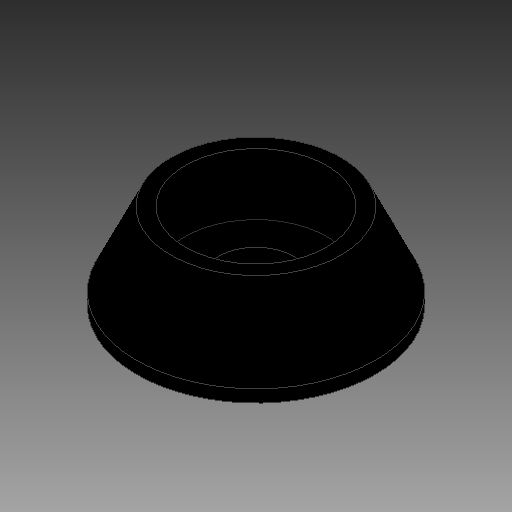
# Autodesk Inventor part: M3 Conical Washer
Saved by Autodesk Inventor 2019 (Build 230136000, 136)
## iProperties
Created: 2018-10-13
Part Number: M3 Conical Washer
Material: Aluminum 6061
Document SubType Name: Modeling
Designer: Ax
Density: 2.7 g/cm^3
Appearance: Anodized - Black
Mass: 0.347814 g
Surface Area: 2.533 cm^2
Volume: 0.12882 cm^3
Author: Ax
Autodesk Inventor part; units mm, degrees
ref_plane "YZ Plane" through (0, 0, 0) normal (1, 0, 0) x (0, 1, 0)
ref_plane "XZ Plane" through (0, 0, 0) normal (0, 1, 0) x (-1, 0, 0)
ref_plane "XY Plane" through (0, 0, 0) normal (0, 0, 1) x (1, 0, 0)
sketch "Sketch1" plane through (0, 0, 0) normal (0, 0, 1) x (1, 0, 0)
  line L0 (2.875, 2.5) -> (2.875, 0)
  line L1 (2.875, 0) -> (1.5, 0)
  line L2 (1.5, 0) -> (1.5, -1)
  line L3 (1.5, -1) -> (4.85, -1)
  line L4 (3.45, 2.5) -> (2.875, 2.5)
  line L5 (0, 0) -> (15.2702, 0) construction
  line L6 (4.85, -1) -> (4.85, -0.5)
  line L7 (4.85, -0.5) -> (3.45, 2.5)
  line L8 (0, -1.7) -> (0, 3.2) projected
  dimension "d0" = 2.875
  dimension "d1" = 1.5
  dimension "d2" = 1
  dimension "d3" = 3.45
  dimension "d4" = 3.5
  dimension "d5" = 4.85
  dimension "d6" = 0.5
  constraints: 16 end point, 2 horizontal, 2 perpendicular, 2 vertical, 1 parallel, 1 point on line
  measures "d0" horizontal distance of L0.start L5.start
  measures "d1" horizontal distance of L5.start L2.end
  measures "d2" distance of L1.end L2.end
  measures "d3" horizontal distance of L5.start L4.start
  measures "d4" vertical distance of L4.start L3.end
  measures "d5" horizontal distance of L5.start L3.end
  measures "d6" distance of L3.end L6.end
revolve "Revolution1" add sketch "Sketch1" angle 360 about axis through (0, -10, 0) along (0, 1, 0)
body "Solid1"
